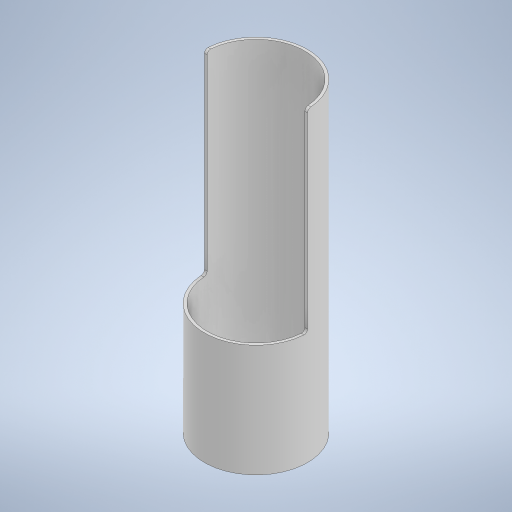
# Autodesk Inventor part: Embellecedor Espejo
Saved by Autodesk Inventor 2024 (Build 280153000, 153)
## iProperties
Created: 2023-08-27
Part Number: Embellecedor Espejo
Material: Genérico
Document SubType Name: Modeling
Designer: sergi
Density: 1 g/cm^3
Appearance: Valor por defecto
Author: sergi
Autodesk Inventor part; units mm, degrees
ref_plane "YZ Plane" through (0, 0, 0) normal (1, 0, 0) x (0, 1, 0)
ref_plane "XZ Plane" through (0, 0, 0) normal (0, 1, 0) x (-1, 0, 0)
ref_plane "XY Plane" through (0, 0, 0) normal (0, 0, 1) x (1, 0, 0)
sketch "Boceto1" plane through (0, 0, 0) normal (0, 1, 0) x (-1, 0, 0)
  circle A0 centre (0, 0) radius 14.35
  circle A1 centre (0, 0) radius 15.15
  dimension "d0" = 28.7
  dimension "d1" = 0.8
  constraints: 2 centre point, 1 coincident
  measures "d0" diameter of A0
  measures "d1" radial gap between concentric circles of A0 A1
extrude "Extrusión1" add sketch "Boceto1" along normal blind 90
sketch "Boceto2" plane through (0, 90, 0) normal (0, 1, 0) x (1, 0, 0)
  circle A0 centre (0, 0) radius 15.15 projected
  circle A1 centre (0, 0) radius 14.35 projected
  line L0 (-15.15, 0) -> (-14.35, 0)
  line L1 (14.35, 0) -> (15.15, 0)
  constraints: 4 end point, 4 point on circle, 1 point on line
extrude "Extrusión2" cut sketch "Boceto2" against normal blind 57 contours A0 L0 A1 L1 picked at (14.5976, -2.3533)
fillet "Empalme1" radius 1 4 edges at (-14.75, 33, 0) (14.75, 33, 0) (-14.75, 90, 0) (14.75, 90, 0)
